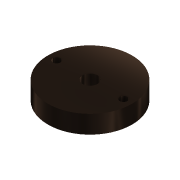
# Autodesk Inventor part: MUSAB6
Saved by Autodesk Inventor 2017 (Build 210142000, 142)
## iProperties
Created: 2017-09-15
Part Number: MUSAB6
Material: Bronze
Document SubType Name: Modeling
Designer: Amer Mohia
Density: 8.47 g/cm^3
Appearance: Bronze - Polished
Author: Amer Mohia
Autodesk Inventor part; units mm, degrees
ref_plane "YZ Plane" through (0, 0, 0) normal (1, 0, 0) x (0, 1, 0)
ref_plane "XZ Plane" through (0, 0, 0) normal (0, 1, 0) x (-1, 0, 0)
ref_plane "XY Plane" through (0, 0, 0) normal (0, 0, 1) x (1, 0, 0)
sketch "Sketch1" plane through (0, 0, 0) normal (0, 0, 1) x (1, 0, 0)
  circle A0 centre (0, 0) radius 7
  dimension "d0" = 14
  constraints: 1 centre point, 1 coincident
  measures "d0" diameter of A0
extrude "Extrusion1" add sketch "Sketch1" along normal blind 3
sketch "Sketch2" plane through (0, 0, 3) normal (0, 0, 1) x (1, 0, 0)
  circle A0 centre (0, 0) radius 1.25
  dimension "d3" = 2.5
  constraints: 1 centre point, 1 coincident
  measures "d3" diameter of A0
extrude "Extrusion2" cut sketch "Sketch2" against normal blind 3
sketch "Sketch3" plane through (0, 0, 3) normal (0, 0, 1) x (1, 0, 0)
  circle A0 centre (-5.575, 0) radius 0.625
  circle A1 centre (0, 0) radius 7 projected
  circle A2 centre (5.575, 0) radius 0.625
  dimension "d6" = 1.25
  dimension "d7" = 1.25
  dimension "d9" = 0.8
  dimension "d10" = 0.8
  dimension "d12" = 9.9
  constraints: 2 centre point
  measures "d6" diameter of A0
  measures "d7" diameter of A2
sketch "Sketch4" plane through (0, 0, 0) normal (0, 1, 0) x (-1, 0, 0)
  line L0 (7, 3) -> (-7, 3) projected
  line L1 (5.5663, 3) -> (5.4, -0.2434)
  line L2 (7, 0) -> (7, 3) projected
  point P0 (0, 0)
  dimension "d13" = 1.6
  constraints: 2 end point, 1 point on line
  measures "d13" distance from line of L2 L1.end
sweep "Sweep1" cut profiles "Sketch3" path "Sketch4" path curves L1 contours A0
sketch "Sketch5" plane through (0, 0, 3) normal (0, 0, 1) x (1, 0, 0)
  circle A0 centre (5.5837, 0) radius 0.625
  circle A1 centre (-5.5663, 0) radius 0.625 projected
  point P0 (0, 0)
  dimension "d16" = 1.25
  dimension "d17" = 9.9
  constraints: 1 centre point
  measures "d16" diameter of A0
sketch "Sketch6" plane through (0, 0, 0) normal (0, 1, 0) x (-1, 0, 0)
  line L0 (-5.575, 2.9594) -> (-5.4, 0)
  line L1 (-7, 0) -> (7, 0) projected
  line L2 (-7, 0) -> (-7, 3) projected
  line L3 (-5.4, 0) -> (-5.4, -0.6456)
  point P0 (0, 0)
  dimension "d18" = 1.425
  dimension "d19" = 1.6
  constraints: 4 end point, 1 point on line, 1 vertical
  measures "d18" distance from line of L2 L0.start
  measures "d19" distance of L0.end L1.start
sweep "Sweep2" cut profiles "Sketch5" path "Sketch6" path curves L0 L3 contours A0
body "Solid1"
